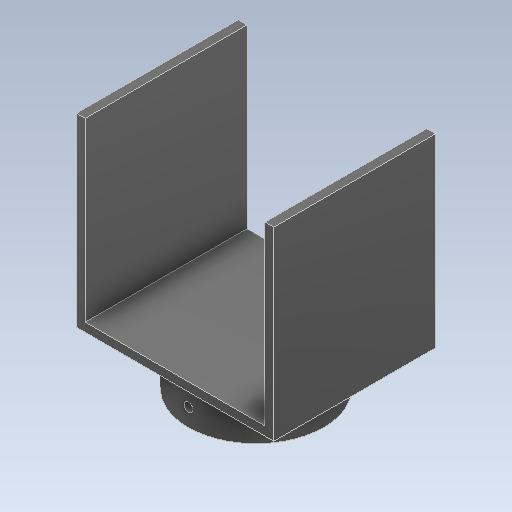
# Autodesk Inventor part: baseatas
Saved by Autodesk Inventor 2025.1 (Build 291241000, 241)
## iProperties
Created: 2024-11-07
Part Number: baseatas
Material: Aluminum 6061
Document SubType Name: Modeling
Designer: ramad
Density: 2.7 g/cm^3
Appearance: Aluminum - Flat
Author: ramad
Autodesk Inventor part; units mm, degrees
ref_plane "YZ Plane" through (0, 0, 0) normal (1, 0, 0) x (0, 1, 0)
ref_plane "XZ Plane" through (0, 0, 0) normal (0, 1, 0) x (-1, 0, 0)
ref_plane "XY Plane" through (0, 0, 0) normal (0, 0, 1) x (1, 0, 0)
sketch "Sketch1" plane through (0, 0, 0) normal (0, 1, 0) x (-1, 0, 0)
  circle A0 centre (0, 0) radius 21
  circle A1 centre (0, 0) radius 23
  dimension "d0" = 42
  dimension "d1" = 2
  constraints: 2 centre point, 1 coincident
  measures "d0" diameter of A0
  measures "d1" radial gap between concentric circles of A0 A1
extrude "Extrusion1" add sketch "Sketch1" along normal blind 15
sketch "Sketch2" plane through (0, 15, 0) normal (0, 1, 0) x (1, 0, 0)
  line L0 (26, -27.5) -> (-26, -27.5)
  line L1 (-26, 27.5) -> (26, 27.5)
  line L2 (26, -27.5) -> (-26, 27.5) construction
  line L3 (-26, -27.5) -> (26, 27.5) construction
  line L4 (-26, 27.5) -> (-29, 27.5)
  line L5 (-29, -27.5) -> (-26, -27.5)
  line L6 (26, 27.5) -> (29, 27.5)
  line L7 (29, -27.5) -> (26, -27.5)
  circle A0 centre (0, 0) radius 11.075
  line L8 (-30.543, 0) -> (-30.543, -27.5)
  line L9 (-30.543, -27.5) -> (-29, -27.5)
  line L10 (-30.543, 0) -> (-30.543, 27.5)
  line L11 (-30.543, 27.5) -> (-29.0865, 27.5)
  line L12 (30.543, 0) -> (30.543, 27.5)
  line L13 (30.543, 27.5) -> (29, 27.5)
  line L14 (30.543, 0) -> (30.543, -27.5)
  line L15 (30.543, -27.5) -> (29, -27.5)
  line L16 (30.543, -27.5) -> (33.543, -27.5)
  line L17 (33.543, -27.5) -> (33.543, 27.5)
  line L18 (33.543, 27.5) -> (30.543, 27.5)
  line L19 (-30.543, 27.5) -> (-33.543, 27.5)
  line L20 (-33.543, 27.5) -> (-33.543, -27.5)
  line L21 (-33.543, -27.5) -> (-30.543, -27.5)
  line L22 (-29.0865, 27.5) -> (-29, 27.5)
  line L23 (30.543, 27.5) -> (33.543, 27.5)
  line L24 (33.543, 27.5) -> (33.543, -27.5)
  line L25 (33.543, -27.5) -> (30.543, -27.5)
  line L26 (30.543, -27.5) -> (30.543, 27.5)
  line L27 (-33.543, 27.5) -> (-30.543, 27.5)
  line L28 (-30.543, 27.5) -> (-30.543, -27.5)
  line L29 (-30.543, -27.5) -> (-33.543, -27.5)
  line L30 (-33.543, -27.5) -> (-33.543, 27.5)
  dimension "d4" = 52
  dimension "d6" = 3
  dimension "d7" = 3
  dimension "d21" = 22.15
  dimension "d23" = 30.543
  dimension "d24" = 3
  constraints: 62 end point, 9 perpendicular, 7 parallel, 7 point on line, 5 horizontal, 3 vertical, 2 midpoint, 1 centre point, 1 coincident, 1 collinear
  measures "d4" distance of L1.start L1.end
  measures "d6" distance of L5.end L5.start
  measures "d7" distance of L7.start L7.end
  measures "d21" diameter of A0
  measures "d23" distance of L12.start point (0, 0)
  measures "d24" distance of L14.end L16.end
extrude "Extrusion2" add sketch "Sketch2" along normal blind 3 contours L0 L5 L9 L8 L10 L11 L22 L4 L1 L6 L13 L12 L14 L15 L7 | A0
sketch "Sketch3" plane through (0, 0, 0) normal (1, 0, 0) x (0, 1, 0)
  circle A0 centre (6, 0) radius 1.5
  line L0 (0, 21) -> (0, -21) projected
  point P0 (0, 0)
  dimension "d14" = 3
  dimension "d15" = 6
  constraints: 1 centre point
  measures "d14" diameter of A0
  measures "d15" distance from line of L0 A0.centre
extrude "Extrusion4" cut sketch "Sketch3" along normal up to surface
pattern_circular "Circular Pattern1" count 8 over 360 about axis through (0, 0, 0) along (0, 1, 0) of "Extrusion4"
extrude "Extrusion5" add sketch "Sketch2" along normal blind 63 contours L14 L12 L18 L17 L16 | L21 L20 L19 L10 L8
equation "\"d23\" = d22"
equation "\"d22\" = 30.543"
body "Solid1"
